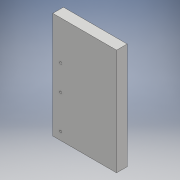
# Autodesk Inventor part: temp back plate
Saved by Autodesk Inventor 2017 (Build 210142000, 142)
## iProperties
Created: 2019-03-03
Part Number: temp back plate
Material: Generic
Document SubType Name: Modeling
Designer: Ben
Density: 1 g/cm^3
Appearance: Default
Author: Ben
Autodesk Inventor part; units mm, degrees
ref_plane "YZ Plane" through (0, 0, 0) normal (1, 0, 0) x (0, 1, 0)
ref_plane "XZ Plane" through (0, 0, 0) normal (0, 1, 0) x (-1, 0, 0)
ref_plane "XY Plane" through (0, 0, 0) normal (0, 0, 1) x (1, 0, 0)
sketch "Sketch1" plane through (0, 0, 0) normal (0, 1, 0) x (-1, 0, 0)
  line L0 (0, 0) -> (60, 0)
  line L1 (60, 0) -> (60, -100)
  line L2 (60, -100) -> (0, -100)
  line L3 (0, -100) -> (0, 0)
  dimension "d0" = 60
  dimension "d1" = 100
  constraints: 8 end point, 2 parallel, 1 horizontal, 1 perpendicular
  measures "d0" distance of L1.end L2.end
  measures "d1" distance of L0.end L1.end
extrude "Extrusion1" add sketch "Sketch1" along normal blind 10
sketch "Sketch2" plane through (0, 10, 0) normal (0, 1, 0) x (1, 0, 0)
  circle A0 centre (-52.5, 60.625) radius 1
  line L0 (0, 100) -> (-60, 100) projected
  line L1 (-60, 100) -> (-60, 0) projected
  point P0 (0, 0)
  dimension "d4" = 2
  dimension "d5" = 39.375
  dimension "d6" = 7.5
  constraints: 1 centre point
  measures "d4" diameter of A0
  measures "d5" distance from line of L0 A0.centre
  measures "d6" distance from line of A0.centre L1
extrude "Extrusion2" cut sketch "Sketch2" against normal blind 10
sketch "Sketch3" plane through (0, 10, 0) normal (0, 1, 0) x (1, 0, 0)
  circle A0 centre (-52.5, 36.625) radius 1
  circle A1 centre (-52.5, 60.625) radius 1 projected
  point P0 (0, 0)
  dimension "d9" = 2
  dimension "d10" = 24
  dimension "d11" = 0
  constraints: 1 centre point
  measures "d9" diameter of A0
  measures "d10" distance of A1.centre A0.centre
  measures "d11" horizontal distance of A1.centre A0.centre
extrude "Extrusion3" cut sketch "Sketch3" against normal blind 10 contours A0
sketch "Sketch4" plane through (0, 10, 0) normal (0, 1, 0) x (1, 0, 0)
  circle A0 centre (-52.5, 92.5) radius 1
  line L0 (0, 100) -> (-60, 100) projected
  line L1 (-60, 100) -> (-60, 0) projected
  point P0 (0, 0)
  dimension "d14" = 2
  dimension "d15" = 7.5
  dimension "d16" = 7.5
  constraints: 1 centre point
  measures "d14" diameter of A0
  measures "d15" distance from line of L0 A0.centre
  measures "d16" distance from line of A0.centre L1
extrude "Extrusion4" cut sketch "Sketch4" against normal blind 10
body "Solid1"
